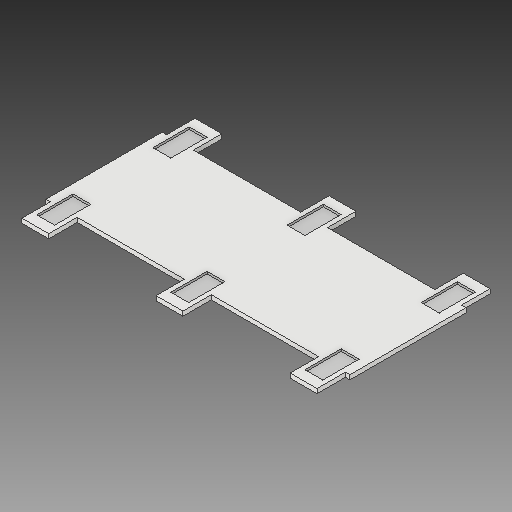
# Autodesk Inventor part: Body_Top
Saved by Autodesk Inventor 2017 (Build 210142000, 142)
## iProperties
Created: 2017-01-25
Part Number: Body_Top
Material: Generic
Document SubType Name: Modeling
Designer: Alexander Miller
Density: 1 g/cm^3
Appearance: Default
Author: Alexander Miller
Autodesk Inventor part; units mm, degrees
ref_plane "YZ Plane" through (0, 0, 0) normal (1, 0, 0) x (0, 1, 0)
ref_plane "XZ Plane" through (0, 0, 0) normal (0, 1, 0) x (-1, 0, 0)
ref_plane "XY Plane" through (0, 0, 0) normal (0, 0, 1) x (1, 0, 0)
sketch "Sketch1" plane through (0, 0, 0) normal (0, 1, 0) x (-1, 0, 0)
  line L0 (-170, 0) -> (-170, -65)
  line L1 (-170, -65) -> (-165, -65)
  line L2 (-165, -65) -> (-165, -96.75)
  line L3 (-165, -96.75) -> (-135, -96.75)
  line L4 (-135, -96.75) -> (-135, -65)
  line L5 (-135, -65) -> (-15, -65)
  line L6 (-15, -65) -> (-15, -96.75)
  line L7 (-15, -96.75) -> (15, -96.75)
  line L8 (15, -96.75) -> (15, -65)
  line L9 (15, -65) -> (135, -65)
  line L10 (135, -65) -> (135, -96.75)
  line L11 (135, -96.75) -> (165, -96.75)
  line L12 (165, -96.75) -> (165, -65)
  line L13 (165, -65) -> (170, -65)
  line L14 (170, -65) -> (170, 0)
  line L15 (210, 0) -> (-210, 0) projected
  line L16 (-170, 0) -> (-170, 65)
  line L17 (-170, 65) -> (-165, 65)
  line L18 (-165, 65) -> (-165, 96.75)
  line L19 (-165, 96.75) -> (-135, 96.75)
  line L20 (-135, 96.75) -> (-135, 65)
  line L21 (-135, 65) -> (-15, 65)
  line L22 (-15, 65) -> (-15, 96.75)
  line L23 (-15, 96.75) -> (15, 96.75)
  line L24 (15, 96.75) -> (15, 65)
  line L25 (15, 65) -> (135, 65)
  line L26 (135, 65) -> (135, 96.75)
  line L27 (135, 96.75) -> (165, 96.75)
  line L28 (165, 96.75) -> (165, 65)
  line L29 (165, 65) -> (170, 65)
  line L30 (170, 65) -> (170, 0)
  point P0 (0, 0)
  point P1 (0, -96.75)
  dimension "d0" = 30
  dimension "d1" = 65
  dimension "d2" = 31.75
  dimension "d3" = 5
  dimension "d4" = 120
  constraints: 60 end point, 18 point on line, 14 symmetric about line, 9 perpendicular, 5 equal length, 2 vertical, 1 horizontal alignment, 1 midpoint, 1 vertical alignment
  measures "d0" distance of L10.end L11.end
  measures "d1" distance of L13.end L14.end
  measures "d2" distance of L11.end L12.end
  measures "d3" distance of L12.end L13.end
  measures "d4" distance of L8.end L9.end
extrude "Extrusion1" add sketch "Sketch1" along normal blind 5
sketch "Sketch2" plane through (0, 5, 0) normal (0, 1, 0) x (1, 0, 0)
  line L0 (-140, 44.75) -> (-160, 44.75)
  line L1 (-160, 44.75) -> (-160, 85.25)
  line L2 (-160, 85.25) -> (-140, 85.25)
  line L3 (-140, 85.25) -> (-140, 44.75)
  line L4 (10, 44.75) -> (-10, 44.75)
  line L5 (-10, 44.75) -> (-10, 85.25)
  line L6 (-10, 85.25) -> (10, 85.25)
  line L7 (10, 85.25) -> (10, 44.75)
  line L8 (160, 44.75) -> (140, 44.75)
  line L9 (140, 44.75) -> (140, 85.25)
  line L10 (140, 85.25) -> (160, 85.25)
  line L11 (160, 85.25) -> (160, 44.75)
  line L12 (-238, 0) -> (238, 0) projected
  line L13 (-140, -44.75) -> (-160, -44.75)
  line L14 (-160, -44.75) -> (-160, -85.25)
  line L15 (-160, -85.25) -> (-140, -85.25)
  line L16 (-140, -85.25) -> (-140, -44.75)
  line L17 (10, -44.75) -> (-10, -44.75)
  line L18 (-10, -44.75) -> (-10, -85.25)
  line L19 (-10, -85.25) -> (10, -85.25)
  line L20 (10, -85.25) -> (10, -44.75)
  line L21 (160, -44.75) -> (140, -44.75)
  line L22 (140, -44.75) -> (140, -85.25)
  line L23 (140, -85.25) -> (160, -85.25)
  line L24 (160, -85.25) -> (160, -44.75)
  line L25 (-135, 96.75) -> (-165, 96.75) projected
  line L26 (-165, 96.75) -> (-165, 65) projected
  line L27 (-15, 96.75) -> (-15, 65) projected
  line L28 (135, 96.75) -> (135, 65) projected
  point P0 (0, 0)
  dimension "d7" = 11.5
  dimension "d8" = 5
  dimension "d9" = 20
  dimension "d10" = 40.5
  dimension "d11" = 5
  dimension "d12" = 5
  constraints: 48 end point, 12 symmetric about line, 6 parallel, 4 point on line, 3 horizontal, 3 perpendicular, 2 collinear, 2 horizontal alignment
  measures "d7" distance between parallel lines of L2 L25
  measures "d8" distance between parallel lines of L1 L26
  measures "d9" distance of L1.end L2.end
  measures "d10" distance of L2.end L0.start
  measures "d11" distance between parallel lines of L27 L5
  measures "d12" distance between parallel lines of L9 L28
extrude "Extrusion2" cut sketch "Sketch2" against normal blind 2.5
equation "\"d0\" = servo_depth + 2 * material_thickness"
equation "\"d1\" = 0.5 * body_width"
equation "\"d2\" = servo_mount_length + 0.5 * servo_width + material_thickness"
equation "\"d4\" = leg_distance"
equation "\"d5\" = material_thickness"
equation "\"d7\" = material_thickness + servo_mount_length"
equation "\"d8\" = material_thickness"
equation "\"d9\" = servo_depth"
equation "\"d10\" = servo_width"
equation "\"d11\" = d8"
equation "\"d12\" = d8"
equation "\"d13\" = 0.5 * material_thickness"
equation "\"material_thickness\" = material_thickness_1"
equation "\"leg_distance\" = leg_distance_1"
equation "\"servo_depth\" = 20"
equation "\"body_width\" = 130"
equation "\"servo_mount_length\" = 6.5"
equation "\"servo_width\" = 40.5"
equation "\"material_thickness_1\" = 5"
equation "\"leg_distance_1\" = 120"
body "Solid1"
